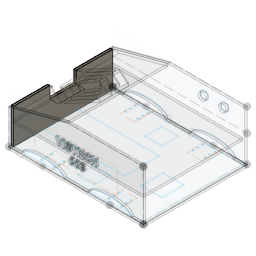
structure_vistech003-v14 (Autodesk Fusion 360 design; units mm, degrees)
Autodesk Fusion 360 part; units mm, degrees
sketch "Sketch1" plane through (0, 0, 0) normal (0, 0, 1) x (1, 0, 0) in component "Base"
  line L0 (-175, -135) -> (175, -135)
  line L1 (175, -135) -> (175, 135)
  line L2 (175, 135) -> (-175, 135)
  line L3 (-175, 135) -> (-175, -135)
  line L4 (-175, 135) -> (175, 135) construction
  line L5 (-169, 129) -> (-169, -129) construction
  line L6 (169, 129) -> (169, -129) construction
  line L7 (-169, -129) -> (169, -129) construction
  line L8 (-169, 129) -> (169, 129) construction
  dimension "d1" = 350
  dimension "d2" = 270
  constraint horizontal L0
  constraint perpendicular L0 L1
  constraint parallel L0 L2
  constraint parallel L1 L3
  constraint perpendicular L3 L4
  constraint vertical L5
  constraint perpendicular L0 L6
  constraint horizontal L7
  constraint perpendicular L1 L8
  measures "d1" distance of L1.end L2.end
  measures "d2" distance of L0.end L1.end
extrude "Extrude1" add sketch "Sketch1" along normal blind 6 makes body 1 in component "Base"
sketch "Sketch2" plane through (0, 0, 6) normal (0, 0, 1) x (-1, 0, 0) in component "Base"
  line L0 (175, -135) -> (175, 135)
  line L1 (175, 135) -> (-175, 135)
  line L2 (-175, 135) -> (-175, -135)
  line L3 (-175, -135) -> (175, -135)
  line L4 (-169, 129) -> (-169, 0) construction
  line L5 (169, 0) -> (169, 129) construction
  line L6 (-107.98, 121.78) -> (-107.98, 84.29) construction
  line L7 (-107.98, 84.29) -> (-70.08, 84.29) construction
  line L8 (-70.08, 84.29) -> (-70.08, 135) construction
  line L9 (-107.98, 135) -> (-70.08, 135) construction
  line L10 (-107.98, 135) -> (-107.98, 121.78) construction
  line L11 (-107.98, 121.78) -> (-107.98, 109.06) construction
  line L12 (-107.98, 109.06) -> (-107.98, 96.34) construction
  circle A0 centre (-104.93, 121.78) radius 1.6
  circle A1 centre (-104.93, 109.06) radius 1.6
  circle A2 centre (-104.93, 96.34) radius 1.6
  circle A3 centre (-73.13, 96.34) radius 1.6
  circle A4 centre (-73.13, 109.06) radius 1.6
  circle A5 centre (-73.13, 121.78) radius 1.6
  line L13 (169, 129) -> (144, 129) construction
  line L14 (104.89, 135) -> (66.99, 135) construction
  line L15 (30.97, 135) -> (30.97, 129) construction
  line L16 (66.99, 135) -> (66.99, 84.29) construction
  line L17 (144, 129) -> (169, 129) construction
  line L18 (66.99, 84.29) -> (104.89, 84.29) construction
  line L19 (104.89, 84.29) -> (104.89, 135) construction
  line L20 (66.99, 135) -> (66.99, 121.78) construction
  line L21 (66.99, 121.78) -> (66.99, 109.06) construction
  line L22 (66.99, 109.06) -> (66.99, 96.34) construction
  circle A6 centre (70.04, 121.78) radius 1.6
  circle A7 centre (70.04, 109.06) radius 1.6
  circle A8 centre (70.04, 96.34) radius 1.6
  circle A9 centre (101.84, 96.34) radius 1.6
  circle A10 centre (101.84, 109.06) radius 1.6
  circle A11 centre (101.84, 121.78) radius 1.6
  line L23 (-169, 0) -> (-169, -129) construction
  line L24 (169, 0) -> (169, -129) construction
  line L25 (-169, -129) -> (-144, -129) construction
  line L26 (-144, -129) -> (-144, -135) construction
  line L27 (-107.98, -135) -> (-107.98, -84.29) construction
  line L28 (-107.98, -84.29) -> (-70.08, -84.29) construction
  line L29 (-70.08, -84.29) -> (-70.08, -135) construction
  line L30 (-30.97, -135) -> (-30.97, -129) construction
  line L31 (-30.97, -129) -> (30.97, -129) construction
  line L32 (30.97, -129) -> (30.97, -135) construction
  line L33 (67.17, -135) -> (67.17, -84.29) construction
  line L34 (67.17, -84.29) -> (105.07, -84.29) construction
  line L35 (105.07, -84.29) -> (105.07, -135) construction
  line L36 (169, -129) -> (144, -129) construction
  line L37 (-107.98, -135) -> (-107.98, -121.78) construction
  line L38 (-107.98, -121.78) -> (-107.98, -109.06) construction
  line L39 (-107.98, -109.06) -> (-107.98, -96.34) construction
  circle A12 centre (-104.93, -121.78) radius 1.6
  circle A13 centre (-104.93, -109.06) radius 1.6
  circle A14 centre (-104.93, -96.34) radius 1.6
  circle A15 centre (-73.13, -96.34) radius 1.6
  circle A16 centre (-73.13, -109.06) radius 1.6
  circle A17 centre (-73.13, -121.78) radius 1.6
  line L40 (67.17, -135) -> (67.17, -121.78) construction
  line L41 (67.17, -121.78) -> (67.17, -109.07) construction
  line L42 (67.17, -109.07) -> (67.17, -96.36) construction
  circle A18 centre (70.22, -96.36) radius 1.6
  circle A19 centre (102.02, -96.36) radius 1.6
  circle A20 centre (70.22, -109.07) radius 1.6
  circle A21 centre (102.02, -109.07) radius 1.6
  circle A22 centre (70.22, -121.78) radius 1.6
  circle A23 centre (102.02, -121.78) radius 1.6
  line L43 (-21.6, -66) -> (21.6, -66)
  line L44 (21.6, -66) -> (21.6, -109)
  line L45 (21.6, -109) -> (-21.6, -109)
  line L46 (-21.6, -109) -> (-21.6, -66)
  line L47 (-21.6, 66) -> (-21.6, 109)
  line L48 (-21.6, 109) -> (21.6, 109)
  line L49 (21.6, 109) -> (21.6, 66)
  line L50 (-21.6, 66) -> (21.6, 66)
  line L51 (-139, 49.8732) -> (-84.92, 49.8732)
  line L52 (-84.92, 49.8732) -> (-84.92, -6.1768)
  line L53 (-84.92, -6.1768) -> (-139, -6.1768)
  line L54 (-139, -6.1768) -> (-139, 49.8732)
  line L55 (169, 50.129) -> (-41, 50.129)
  line L56 (-41, 50.129) -> (-41, -39.871)
  line L57 (-41, -39.871) -> (169, -39.871)
  line L58 (169, -39.871) -> (169, 50.129)
  line L59 (-169, 129) -> (-175, 129) construction
  line L60 (-169, -129) -> (-175, -129) construction
  line L61 (169, -129) -> (175, -129) construction
  line L62 (169, 129) -> (175, 129) construction
  line L63 (-175, 129) -> (-169, 129)
  line L64 (-169, 129) -> (-169, -129)
  line L65 (-169, -129) -> (-175, -129)
  line L66 (-175, 129) -> (-175, -129)
  line L67 (169, 129) -> (175, 129)
  line L68 (169, 129) -> (169, -129)
  line L69 (169, -129) -> (175, -129)
  line L70 (-175, -135) -> (175, -135)
  line L71 (144, -129) -> (144, -135) construction
  line L72 (175, -129) -> (175, -135)
  line L73 (175, -135) -> (-175, -135)
  line L74 (-175, -135) -> (-175, -129)
  line L75 (-169, -129) -> (169, -129)
  line L76 (-144, 129) -> (-144, 135) construction
  line L77 (-169, 129) -> (-144, 129) construction
  line L78 (-30.97, 129) -> (-30.97, 135) construction
  line L79 (-30.97, 129) -> (30.97, 129) construction
  line L80 (144, 129) -> (144, 135) construction
  line L81 (175, 129) -> (175, 135)
  line L82 (175, 135) -> (-175, 135)
  line L83 (-175, 129) -> (-175, 135)
  line L84 (-169, 129) -> (169, 129)
  point P0 (-175, -135)
  dimension "d20" = 25
  dimension "d23" = 37.9
  dimension "d27" = 13.22
  dimension "d28" = 12.72
  dimension "d29" = 12.72
  dimension "d30" = 3.05
  dimension "d32" = 3.05
  dimension "d34" = 3.05
  dimension "d36" = 3.2
  dimension "d37" = 3.2
  dimension "d38" = 3.2
  dimension "d39" = 3.2
  dimension "d40" = 3.2
  dimension "d41" = 3.2
  dimension "d42" = 25
  dimension "d44" = 36.02
  dimension "d45" = 50.71
  dimension "d46" = 37.9
  dimension "d47" = 13.22
  dimension "d48" = 12.72
  dimension "d49" = 12.72
  dimension "d57" = 3.2
  dimension "d58" = 3.2
  dimension "d59" = 3.2
  dimension "d60" = 3.2
  dimension "d61" = 3.2
  dimension "d62" = 3.2
  dimension "d66" = 25
  dimension "d67" = 36.02
  dimension "d68" = 50.71
  dimension "d69" = 37.9
  dimension "d70" = 39.11
  dimension "d72" = 61.94
  dimension "d73" = 36.2
  dimension "d74" = 50.71
  dimension "d75" = 37.9
  dimension "d78" = 25
  dimension "d79" = 13.22
  dimension "d80" = 12.72
  dimension "d81" = 12.72
  dimension "d82" = 3.05
  dimension "d83" = 3.05
  dimension "d84" = 3.05
  dimension "d88" = 3.2
  dimension "d89" = 3.2
  dimension "d90" = 3.2
  dimension "d91" = 3.2
  dimension "d92" = 3.2
  dimension "d93" = 3.2
  dimension "d94" = 13.22
  dimension "d95" = 12.71
  dimension "d96" = 12.71
  dimension "d97" = 3.05
  dimension "d99" = 3.05
  dimension "d101" = 3.05
  dimension "d103" = 3.2
  dimension "d104" = 3.2
  dimension "d105" = 3.2
  dimension "d106" = 3.2
  dimension "d107" = 3.2
  dimension "d108" = 3.2
  dimension "d116" = 43.2
  dimension "d124" = 43.2
  dimension "d125" = 43
  dimension "d130" = 43.2
  dimension "d133" = 43
  dimension "d139" = 54.08
  dimension "d140" = 56.05
  dimension "d143" = 210
  dimension "d144" = 90
  constraint perpendicular L1 L4
  constraint perpendicular L6 L7
  constraint coincident L1 L8.end
  constraint perpendicular L1 L8
  constraint perpendicular L1 L10
  constraint parallel L6 L11
  constraint parallel L6 L12
  constraint perpendicular L0 L13
  constraint perpendicular L16 L18
  constraint vertical L19
  constraint parallel L16 L21
  constraint parallel L16 L22
  constraint perpendicular L3 L23
  constraint perpendicular L23 L25
  constraint coincident L3 L26.end
  constraint perpendicular L3 L26
  constraint coincident L3 L27.start
  constraint perpendicular L27 L28
  constraint coincident L3 L29.end
  constraint perpendicular L3 L29
  constraint perpendicular L30 L31
  constraint coincident L3 L32.end
  constraint perpendicular L3 L32
  constraint perpendicular L33 L34
  constraint coincident L3 L35.end
  constraint perpendicular L3 L35
  constraint perpendicular L24 L36
  constraint perpendicular L3 L37
  constraint parallel L27 L38
  constraint parallel L27 L39
  constraint perpendicular L3 L40
  constraint parallel L33 L41
  constraint parallel L33 L42
  constraint perpendicular L43 L44
  constraint perpendicular L44 L45
  constraint perpendicular L49 L50
  constraint horizontal L51
  constraint vertical L52
  constraint horizontal L53
  constraint vertical L54
  constraint horizontal L55
  constraint vertical L56
  constraint horizontal L57
  constraint vertical L58
  constraint coincident L5 L55.start
  constraint coincident L2 L59.end
  constraint perpendicular L2 L59
  constraint coincident L2 L60.end
  constraint perpendicular L2 L60
  constraint coincident L0 L61.end
  constraint perpendicular L0 L61
  constraint coincident L0 L62.end
  constraint perpendicular L0 L62
  constraint perpendicular L36 L68
  constraint coincident L3 L71.end
  constraint perpendicular L3 L71
  constraint coincident L0.start L3.end
  constraint coincident P0 L2.end
  constraint perpendicular L24 L75
  constraint coincident L1 L76.end
  constraint perpendicular L1 L76
  constraint perpendicular L76 L77
  constraint coincident L1 L78.end
  constraint perpendicular L1 L78
  constraint perpendicular L15 L79
  constraint coincident L1 L80.end
  constraint perpendicular L1 L80
  constraint coincident L0.end L1.start
  constraint coincident L1.end L2.start
  constraint perpendicular L5 L84
  measures "d20" distance of L4.start L76.start
  measures "d23" distance of L6.end L7.end
  measures "d27" distance of L9.start L6.start
  measures "d28" distance of L6.start L11.end
  measures "d29" distance of L11.end L12.end
  measures "d30" distance of L12.end A2.centre
  measures "d32" distance of L11.end A1.centre
  measures "d34" distance of L6.start A0.centre
  measures "d36" diameter of A0
  measures "d37" diameter of A1
  measures "d38" diameter of A2
  measures "d39" diameter of A3
  measures "d40" diameter of A4
  measures "d41" diameter of A5
  measures "d42" distance of L5.end L13.end
  measures "d44" distance of L15.start L14.end
  measures "d45" distance of L14.end L16.end
  measures "d46" distance of L16.end L18.end
  measures "d47" distance of L14.end L20.end
  measures "d48" distance of L20.end L21.end
  measures "d49" distance of L21.end L22.end
  measures "d57" diameter of A6
  measures "d58" diameter of A7
  measures "d59" diameter of A8
  measures "d60" diameter of A9
  measures "d61" diameter of A10
  measures "d62" diameter of A11
  measures "d66" distance of L23.end L25.end
  measures "d67" distance of L26.end L27.start
  measures "d68" distance of L27.start L27.end
  measures "d69" distance of L27.end L28.end
  measures "d70" distance of L29.end L30.start
  measures "d72" distance of L30.end L31.end
  measures "d73" distance of L32.end L33.start
  measures "d74" distance of L33.start L33.end
  measures "d75" distance of L33.end L34.end
  measures "d78" distance of L24.end L36.end
  measures "d79" distance of L27.start L37.end
  measures "d80" distance of L37.end L38.end
  measures "d81" distance of L38.end L39.end
  measures "d82" distance of L37.end A12.centre
  measures "d83" distance of L38.end A13.centre
  measures "d84" distance of L39.end A14.centre
  measures "d88" diameter of A12
  measures "d89" diameter of A13
  measures "d90" diameter of A14
  measures "d91" diameter of A15
  measures "d92" diameter of A16
  measures "d93" diameter of A17
  measures "d94" distance of L33.start L40.end
  measures "d95" distance of L40.end L41.end
  measures "d96" distance of L41.end L42.end
  measures "d97" distance of L40.end A22.centre
  measures "d99" distance of L41.end A20.centre
  measures "d101" distance of L42.end A18.centre
  measures "d103" diameter of A18
  measures "d104" diameter of A19
  measures "d105" diameter of A20
  measures "d106" diameter of A21
  measures "d107" diameter of A22
  measures "d108" diameter of A23
  measures "d116" distance of L49.end L47.start
  measures "d124" distance of L43.start L43.end
  measures "d125" distance of L43.end L44.end
  measures "d130" distance of L44.end L45.end
  measures "d133" distance of L47.start L47.end
  measures "d139" distance of L51.start L51.end
  measures "d140" distance of L51.start L53.end
  measures "d143" distance of L55.start L55.end
  measures "d144" distance of L55.start L57.end
extrude "Extrude3" add sketch "Sketch2" along normal blind 130.5 separate body contours L2 L63 L64 L65 L66 makes body 2 in component "Back_panel"
sketch "Sketch5" plane through (175, 0, 0) normal (1, 0, 0) x (0, 1, 0) in component "Back_panel"
  line L0 (-129, 6) -> (129, 6)
  line L1 (129, 6) -> (129, 136.5)
  line L2 (129, 136.5) -> (-129, 136.5)
  line L3 (-129, 136.5) -> (-129, 6)
  line L4 (-129, 76.5) -> (-45, 76.5) construction
  circle A0 centre (-45, 106.5) radius 7.025
  circle A1 centre (-55, 36.5) radius 7.025
  circle A2 centre (55, 36.5) radius 7.025
  line L5 (-45, 76.5) -> (129, 76.5) construction
  dimension "d187" = 14.05
  dimension "d191" = 14.05
  dimension "d192" = 14.05
  constraint coincident L3 L4.start
  constraint perpendicular L1 L4
  constraint coincident L1 L5.end
  constraint perpendicular L1 L5
  measures "d187" diameter of A0
  measures "d191" diameter of A1
  measures "d192" diameter of A2
extrude "Extrude4" cut sketch "Sketch5" along normal through all and the other way through all contours A0 | A1 | A2 bodies 2 in component "Back_panel"
sketch "Sketch2 (2)" plane through (0, 0, 6) normal (0, 0, 1) x (-1, 0, 0) in component "Right_panel"
  line L0 (175, -135) -> (-175, -135)
  line L1 (-169, -129) -> (169, -129)
  line L2 (-169, -129) -> (-175, -129)
  line L3 (-175, -135) -> (-175, -129)
  line L4 (169, -129) -> (175, -129)
  line L5 (175, -129) -> (175, -135)
extrude "Extrude1'" add sketch "Sketch2 (2)" along normal blind 130.5 separate body makes body 3 in component "Right_panel"
sketch "Sketch3" plane through (0, 135, 0) normal (0, 1, 0) x (-1, 0, 0) in component "Right_panel"
  line L0 (-175, 6) -> (175, 6)
  line L1 (175, 6) -> (175, 136.5)
  line L2 (175, 136.5) -> (-175, 136.5)
  line L3 (-175, 136.5) -> (-175, 6)
  line L4 (-175, 6) -> (-169, 6) construction
  line L5 (-169, 6) -> (-144, 6) construction
  line L6 (-144, 6) -> (-87.485, 6) construction
  line L7 (175, 6) -> (144, 6) construction
  line L8 (144, 6) -> (87.485, 6) construction
  ellipse E0 centre (87.485, 6) end of major axis (144, 6) minor radius 20.25 (144, 6) -> (30.97, 6) ccw
  line L9 (-175, 136.5) -> (25, 136.5) construction
  line L10 (175, 6) -> (175, 96.5) construction
  line L11 (175, 96.5) -> (25, 136.5)
  ellipse E1 centre (-87.485, 6) end of major axis (-144, 6) minor radius 20.25 (-30.97, 6) -> (-144, 6) ccw
  line L12 (175, 6) -> (175, 76.5) construction
  line L13 (175, 76.5) -> (-175, 76.5) construction
  circle A0 centre (-116.7012, 106.5) radius 10.055
  circle A1 centre (-63.4141, 106.5) radius 10.055
  dimension "d198" = 56.515
  dimension "d201" = 56.515
  dimension "d202" = 40.5
  dimension "d203" = 200
  dimension "d204" = 90.5
  dimension "d205" = 40.5
  dimension "d207" = 70.5
  dimension "d208" = 20.11
  dimension "d209" = 20.11
  constraint coincident L0.start L3.end
  constraint perpendicular L3 L4
  constraint perpendicular L3 L5
  constraint parallel L0 L6
  constraint coincident L0.end L1.start
  constraint perpendicular L1 L7
  constraint parallel L0 L8
  constraint coincident L8.end E0.centre
  constraint coincident L2.end L3.start
  constraint perpendicular L3 L9
  constraint perpendicular L7 L10
  constraint coincident L6.end E1.centre
  constraint perpendicular L7 L12
  constraint coincident L3 L13.end
  constraint perpendicular L3 L13
  measures "d198" distance of L5.end L6.end
  measures "d201" distance of L7.end L8.end
  measures "d203" distance of L2.end L9.end
  measures "d204" distance of L0.end L10.end
  measures "d207" distance of L0.end L12.end
  measures "d208" diameter of A0
  measures "d209" diameter of A1
extrude "Extrude2" cut sketch "Sketch3" along normal through all and the other way through all contours L0 E1 | L1 L2 L11 | L0 E0 bodies 3 in component "Right_panel"
extrude "Extrude4'" cut sketch "Sketch3" along normal through all and the other way through all contours A0 | A1 bodies 3 in component "Right_panel"
sketch "Sketch1 (2)" plane through (0, 0, 6) normal (0, 0, 1) x (-1, 0, 0) in component "Left_panel"
extrude "Extrude1''" add sketch "Sketch2" along normal blind 130.5 separate body contours L0 L1 L2 L63 L67 L81 L82 L83 L84 makes body 4 in component "Left_panel"
sketch "Sketch2 (3)" plane through (0, -135, 0) normal (0, -1, 0) x (1, 0, 0) in component "Left_panel"
  line L0 (-175, 6) -> (175, 6)
  line L1 (175, 6) -> (175, 136.5)
  line L2 (175, 136.5) -> (-175, 136.5)
  line L3 (-175, 136.5) -> (-175, 6)
  line L4 (175, 6) -> (175, 136.5) construction
  line L5 (175, 136.5) -> (-25, 136.5) construction
  line L6 (-175, 6) -> (-175, 96.5) construction
  line L7 (-175, 96.5) -> (-25, 136.5)
  line L8 (-108.1193, 33.6737) -> (107.6013, 36.6083) construction
  line L9 (107.6013, 36.6083) -> (106.7287, 100.747) construction
  line L10 (106.7287, 100.747) -> (-108.9919, 97.8123) construction
  line L11 (-108.9919, 97.8123) -> (-108.1193, 33.6737) construction
  line L12 (175, 6) -> (144, 6) construction
  line L13 (144, 6) -> (87.485, 6) construction
  ellipse E0 centre (87.485, 6) end of major axis (144, 6) minor radius 20 (144, 6) -> (30.97, 6) ccw
  line L14 (30.97, 6) -> (-30.97, 6) construction
  line L15 (-30.97, 6) -> (-87.485, 6) construction
  ellipse E1 centre (-87.485, 6) end of major axis (-30.97, 6) minor radius 20 (-30.97, 6) -> (-144, 6) ccw
  dimension "d215" = 200
  dimension "d216" = 90.5
  dimension "d218" = 18
  dimension "d254" = 31
  dimension "d255" = 56.515
  dimension "d256" = 40
  dimension "d257" = 61.94
  dimension "d258" = 56.515
  dimension "d259" = 40
  text T0 "VISTECH\n003" font "Arial" height 18 bold align centre middle in box 215.7405 x 64.1446 at (-108.1193, 33.6737) x (0.999907, 0.013603) y (-0.013603, 0.999907) spacing 1 kerned
  constraint coincident L0.end L1.start
  constraint coincident L1.end L2.start
  constraint perpendicular L1 L5
  constraint coincident L0.start L3.end
  constraint perpendicular L0 L6
  constraint perpendicular L1 L12
  constraint parallel L0 L13
  constraint coincident L13.end E0.centre
  constraint parallel L0 L14
  constraint parallel L0 L15
  constraint coincident L15.end E1.centre
  measures "d215" distance of L1.end L5.end
  measures "d216" distance of L0.start L6.end
  measures "d254" distance of L0.end L12.end
  measures "d255" distance of L12.end L13.end
  measures "d257" distance of L14.start L14.end
  measures "d258" distance of L14.end L15.end
extrude "Extrude2'" cut sketch "Sketch2 (3)" along normal through all and the other way through all contours L2 L3 L7 bodies 4 in component "Left_panel"
extrude "Extrude5" cut sketch "Sketch2 (3)" against normal blind 10 text T0 bodies 4 makes body 5 at (-14.3265, -135, 51.7066) makes body 6 at (-0.3428, -135, 51.8968) in component "Left_panel"
sketch "Sketch1 (3)" plane through (0, 0, 6) normal (0, 0, 1) x (-1, 0, 0) in component "Front_panel"
extrude "Extrude1'''" add sketch "Sketch2" along normal blind 90.5 separate body contours L0 L58 L67 L68 L69 makes body 7 in component "Front_panel"
sketch "Sketch4" plane through (0, 129, 0) normal (0, -1, 0) x (1, 0, 0) in component "Right_panel"
  circle A0 centre (116.7012, 106.5) radius 10.055
  circle A1 centre (63.4141, 106.5) radius 10.055
  ellipse E0 centre (87.485, 6) end of major axis (144, 6) minor radius 20.25 (144, 6) -> (30.97, 6) ccw
  line L0 (144, 6) -> (175, 6)
  line L1 (175, 6) -> (175, 136.5)
  line L2 (175, 136.5) -> (-25, 136.5)
  line L3 (-25, 136.5) -> (-175, 96.5)
  line L4 (-175, 96.5) -> (-175, 6)
  line L5 (-175, 6) -> (-144, 6)
  ellipse E1 centre (-87.485, 6) end of major axis (-144, 6) minor radius 20.25 (-30.97, 6) -> (-144, 6) ccw
  line L6 (-30.97, 6) -> (30.97, 6)
  line L7 (-25, 136.5) -> (-175, 96.5) construction
  line L8 (-175, 96.5) -> (-151.7137, 96.5)
  line L9 (-130.1446, 102.2518) -> (-151.7137, 96.5)
  line L10 (-25, 136.5) -> (-25, 130.2903)
  line L11 (-130.1446, 102.2518) -> (-25, 130.2903)
  line L12 (-169, 60) -> (169, 60)
  line L13 (169, 66) -> (-169, 66)
  line L14 (-169, 60) -> (-169, 66)
  line L15 (169, 66) -> (169, 60)
  line L16 (-25, 130.2903) -> (169, 130.2903)
  line L17 (169, 130.2903) -> (169, 136.2903)
  line L18 (169, 136.2903) -> (-25, 136.5)
  line L19 (-25, 136.5) -> (-25, 130.2903)
  dimension "d269" = 6
  constraint coincident L2.end L3.start
  constraint coincident L3.end L4.start
  constraint perpendicular L4 L8
  constraint vertical L10
  constraint parallel L9 L11
  constraint horizontal L12
  constraint perpendicular L13 L14
  constraint perpendicular L12 L15
  constraint perpendicular L1 L16
  constraint perpendicular L2 L17
  measures "d269" distance of L16.end L17.end
sketch "Sketch1 (4)" plane through (0, 129, 0) normal (0, -1, 0) x (1, 0, 0) in component "window_panel"
extrude "Extrude1''''" add sketch "Sketch4" along normal up to surface (258 mm away) separate body contours L3 L8 L9 L10 L11 L19 makes body 8 in component "window_panel"
sketch "Sketch2 (4)" plane through (-35.6432, 0, 133.6618) normal (-0.257663, 0, 0.966235) x (0, -1, 0) in component "window_panel"
  line L0 (129, -144.2267) -> (129, 11.0151)
  line L1 (129, 11.0151) -> (-129, 11.0151)
  line L2 (-129, 11.0151) -> (-129, -144.2267)
  line L3 (-129, -144.2267) -> (129, -144.2267)
  line L4 (-72.1688, -61.6059) -> (-37.5278, -1.6059)
  line L5 (-37.5278, -1.6059) -> (-5, -1.6059)
  line L6 (-5, -1.6059) -> (-5, -16.6059)
  line L7 (-28.8675, -16.6059) -> (-5, -16.6059)
  line L8 (-28.8675, -16.6059) -> (-54.8482, -61.6059)
  line L9 (-54.8482, -61.6059) -> (-72.1688, -61.6059)
  line L10 (-37.5277, -61.6059) -> (-20.2073, -31.6059)
  line L11 (-5, -31.6059) -> (-20.2073, -31.6059)
  line L12 (-5, -31.6059) -> (-5, -46.6059)
  line L13 (-11.547, -46.6059) -> (-5, -46.6059)
  line L14 (-11.547, -46.6059) -> (-20.2072, -61.6059)
  line L15 (-37.5277, -61.6059) -> (-20.2072, -61.6059)
  line L16 (5, -31.6059) -> (5, -46.6059)
  line L17 (5, -31.6059) -> (20.2073, -31.6059)
  line L18 (11.547, -46.6059) -> (5, -46.6059)
  line L19 (11.547, -46.6059) -> (20.2072, -61.6059)
  line L20 (37.5277, -61.6059) -> (20.2073, -31.6059)
  line L21 (20.2072, -61.6059) -> (37.5277, -61.6059)
  line L22 (54.8482, -61.6059) -> (72.1688, -61.6059)
  line L23 (5, -16.6059) -> (5, -1.6059)
  line L24 (5, -16.6059) -> (28.8675, -16.6059)
  line L25 (37.5278, -1.6059) -> (5, -1.6059)
  line L26 (28.8675, -16.6059) -> (54.8482, -61.6059)
  line L27 (72.1688, -61.6059) -> (37.5278, -1.6059)
  line L28 (-5, -116.6059) -> (-5, -131.6059)
  line L29 (-72.1688, -71.6059) -> (-54.8483, -71.6059)
  line L30 (-28.8675, -116.6059) -> (-54.8483, -71.6059)
  line L31 (-72.1688, -71.6059) -> (-37.5278, -131.6059)
  line L32 (-37.5278, -131.6059) -> (-5, -131.6059)
  line L33 (-5, -116.6059) -> (-28.8675, -116.6059)
  line L34 (-5, -101.6059) -> (-5, -86.6059)
  line L35 (-20.2073, -71.6059) -> (-37.5278, -71.6059)
  line L36 (-11.547, -86.6059) -> (-20.2073, -71.6059)
  line L37 (-37.5278, -71.6059) -> (-20.2073, -101.6059)
  line L38 (-11.547, -86.6059) -> (-5, -86.6059)
  line L39 (-5, -101.6059) -> (-20.2073, -101.6059)
  line L40 (5, -86.6059) -> (5, -101.6059)
  line L41 (20.2073, -71.6059) -> (37.5278, -71.6059)
  line L42 (20.2073, -101.6059) -> (5, -101.6059)
  line L43 (5, -86.6059) -> (11.547, -86.6059)
  line L44 (20.2073, -101.6059) -> (37.5278, -71.6059)
  line L45 (11.547, -86.6059) -> (20.2073, -71.6059)
  line L46 (54.8483, -71.6059) -> (72.1688, -71.6059)
  line L47 (5, -131.6059) -> (5, -116.6059)
  line L48 (5, -116.6059) -> (28.8675, -116.6059)
  line L49 (37.5278, -131.6059) -> (5, -131.6059)
  line L50 (28.8675, -116.6059) -> (54.8483, -71.6059)
  line L51 (72.1688, -71.6059) -> (37.5278, -131.6059)
  point P0 (0, -66.6059)
  point P1 (0, -66.6059)
  point P2 (0, -66.6059)
  point P3 (0, -66.6059)
  constraint perpendicular L16 L17
  constraint perpendicular L16 L18
  constraint parallel L19 L20
  constraint horizontal L21
  constraint horizontal L22
  constraint perpendicular L23 L24
  constraint perpendicular L23 L25
  constraint parallel L26 L27
  constraint perpendicular L28 L29
  constraint parallel L30 L31
  constraint perpendicular L28 L32
  constraint perpendicular L28 L33
  constraint perpendicular L34 L35
  constraint parallel L36 L37
  constraint perpendicular L34 L38
  constraint perpendicular L34 L39
  constraint perpendicular L40 L41
  constraint perpendicular L40 L42
  constraint perpendicular L40 L43
  constraint parallel L44 L45
  constraint horizontal L46
  constraint perpendicular L47 L48
  constraint perpendicular L47 L49
  constraint parallel L50 L51
extrude "Extrude2''" cut sketch "Sketch2 (4)" along normal mid plane 12 contours L4 L5 L6 L7 L8 L9 | L10 L11 L12 L13 L14 L15 | L16 L17 L18 L19 L20 L21 | L22 L23 L24 L25 L26 L27 | L28 L29 L30 L31 L32 L33 | L34 L35 L36 L37 L38 L39 | L40 L41 L42 L43 L44 L45 | L46 L47 L48 L49 L50 L51 bodies 8 in component "window_panel"
sketch "Sketch1 (5)" plane through (0, 129, 0) normal (0, -1, 0) x (1, 0, 0) in component "Level_panel"
  line L0 (-169, 60) -> (169, 60)
  line L1 (-169, 60) -> (-169, 66)
  line L2 (169, 66) -> (-169, 66)
  line L3 (169, 66) -> (169, 60)
extrude "Extrude1'''''" add sketch "Sketch1 (5)" along normal blind 258 separate body makes body 9 in component "Level_panel"
extrude "Extrude8" cut sketch "Sketch2 (3)" against normal blind 20 contours L0 E1 bodies 4 in component "Left_panel"
extrude "Extrude9" cut sketch "Sketch2 (3)" against normal blind 30 contours L0 E0 bodies 4 in component "Left_panel"
sketch "Sketch1 (6)" plane through (0, 129, 0) normal (0, -1, 0) x (1, 0, 0) in component "Top_panel"
extrude "Extrude1''''''" add sketch "Sketch4" along normal up to surface (258 mm away) separate body contours L10 L16 L17 L18 L19 makes body 10 in component "Top_panel"
sketch "Sketch2 (5)" plane through (-169, 0, 0) normal (1, 0, 0) x (0, 1, 0) in component "Front_panel"
  line L0 (-129, 6) -> (129, 6)
  line L1 (129, 6) -> (129, 96.5)
  line L2 (129, 96.5) -> (-129, 96.5)
  line L3 (-129, 96.5) -> (-129, 6)
  line L4 (0, 96.5) -> (0, 98.9885) construction
  line L5 (-34.2, 65.9885) -> (-34.2, 105.9885)
  line L6 (-34.2, 65.9885) -> (34.2, 65.9885)
  line L7 (-34.2, 105.9885) -> (34.2, 105.9885)
  line L8 (34.2, 65.9885) -> (34.2, 105.9885)
  dimension "d276" = 40
  dimension "d277" = 68.4
  constraint coincident L2 L4.start
  constraint perpendicular L5 L6
  constraint perpendicular L5 L7
  constraint perpendicular L7 L8
  measures "d276" distance of L5.start L5.end
  measures "d277" distance of L5.start L6.end
extrude "Extrude2'''" cut sketch "Sketch2 (5)" along normal up to surface (-6 mm away) and the other way blind -22 contours L2 L5 L7 L8 | L2 L5 L6 L8 bodies 7 in component "Front_panel"
extrude "Extrude2''''" cut sketch "Sketch2 (5)" along normal up to surface (-6 mm away) and the other way blind -22 contours L2 L5 L7 L8 | L2 L5 L6 L8 bodies 9 in component "Level_panel"
extrude "Extrude3'" cut sketch "Sketch2 (5)" along normal up to surface (-6 mm away) and the other way blind -22 contours L2 L5 L7 L8 | L2 L5 L6 L8 bodies 8 in component "window_panel"
extrude "Extrude7" [suppressed] in component "Left_panel"
extrude "Extrude6" [suppressed] in component "Left_panel"
extrude "Extrude4''" [suppressed] in component "Left_panel"
extrude "Extrude3''" [suppressed] in component "Left_panel"
extrude "Extrude3'''" [suppressed] in component "Right_panel"
extrude "Extrude2'''''" [suppressed] in component "Base"
extrude "Extrude4'''" [suppressed] in component "Base"
extrude "Extrude5'" [suppressed] in component "Base"
extrude "Extrude6'" [suppressed] in component "Base"
extrude "Extrude8'" [suppressed] in component "Base"
extrude "Extrude11" [suppressed] in component "Base"
extrude "Extrude14" [suppressed] in component "Base"
extrude "Extrude15" [suppressed] in component "Base"
extrude "Extrude13" [suppressed] in component "Base"
extrude "Extrude12" [suppressed] in component "Base"
extrude "Extrude10" [suppressed] in component "Base"
extrude "Extrude9'" [suppressed] in component "Base"
extrude "Extrude7'" [suppressed] in component "Base"
extrude "Extrude3''''" [suppressed] in component "Base"
extrude "Extrude17" [suppressed] in component "Base"
extrude "Extrude19" [suppressed] in component "Base"
extrude "Extrude20" [suppressed] in component "Base"
extrude "Extrude21" [suppressed] in component "Base"
extrude "Extrude22" [suppressed] in component "Base"
extrude "Extrude23" [suppressed] in component "Base"
extrude "Extrude24" [suppressed] in component "Base"
extrude "Extrude25" [suppressed] in component "Base"
extrude "Extrude26" [suppressed] in component "Base"
sketch "Sketch2 (6)" plane through (0, 0, 6) normal (0, 0, 1) x (-1, 0, 0) in component "Back_panel"
  line L0 (-175, 129) -> (-169, 129)
  line L1 (-169, 129) -> (-169, -129)
  line L2 (-175, 129) -> (-175, -129)
  line L3 (-169, -129) -> (-175, -129)
extrude "Extrude1'''''''" [suppressed] in component "Back_panel"
sketch "Sketch3 (2)" plane through (175, 0, 0) normal (1, 0, 0) x (0, 1, 0) in component "Back_panel"
  line L0 (-129, 6) -> (129, 6)
  line L1 (129, 6) -> (129, 136)
  line L2 (129, 136) -> (-129, 136)
  line L3 (-129, 136) -> (-129, 6)
  line L4 (-129, 76.5) -> (129, 76.5) construction
  circle A0 centre (-41.7149, 88.306) radius 7.025
  circle A1 centre (-68.4885, 36) radius 7.025
  circle A2 centre (71.8486, 36) radius 7.025
  line L5 (0, 6) -> (0, 36) construction
  dimension "d176" = 14.05
  dimension "d177" = 30
  dimension "d178" = 14.05
  dimension "d179" = 14.05
  constraint coincident L3 L4.start
  constraint coincident L1 L4.end
  constraint perpendicular L1 L4
  constraint midpoint L0 L5.start
  constraint perpendicular L0 L5
  measures "d176" diameter of A0
  measures "d177" distance of L5.start L5.end
  measures "d178" diameter of A2
  measures "d179" diameter of A1
extrude "Extrude2''''''" [suppressed] in component "Back_panel"
extrude "Extrude18" [suppressed] in component "Base"
extrude "Extrude16" [suppressed] in component "Base"
component "Base" placed x (1, 0, 0) y (0, 1, 0) z (0, 0, 1) at (0, 0, 0)
component "Back_panel" placed x (1, 0, 0) y (0, 1, 0) z (0, 0, 1) at (0, 0, 0)
component "Right_panel" placed x (1, 0, 0) y (0, 1, 0) z (0, 0, 1) at (0, 0, 0)
component "Left_panel" placed x (1, 0, 0) y (0, 1, 0) z (0, 0, 1) at (0, 0, 0)
component "Front_panel" placed x (1, 0, 0) y (0, 1, 0) z (0, 0, 1) at (0, 0, 0)
component "Level_panel" placed x (1, 0, 0) y (0, 1, 0) z (0, 0, 1) at (0, 0, 0)
component "Top_panel" placed x (1, 0, 0) y (0, 1, 0) z (0, 0, 1) at (0, 0, 0)
component "window_panel" placed x (1, 0, 0) y (0, 1, 0) z (0, 0, 1) at (0, 0, 0)
